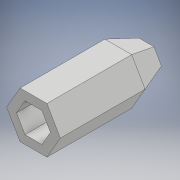
# Autodesk Inventor part: Pieza1
Saved by Autodesk Inventor 2018.2 (Build 222227000, 227)
## iProperties
Created: 2018-01-25
Part Number: Pieza1
Material: Genérico
Document SubType Name: Modeling
Designer: alber
Density: 1 g/cm^3
Appearance: Valor por defecto
Author: alber
Autodesk Inventor part; units mm, degrees
ref_plane "YZ Plane" through (0, 0, 0) normal (1, 0, 0) x (0, 1, 0)
ref_plane "XZ Plane" through (0, 0, 0) normal (0, 1, 0) x (-1, 0, 0)
ref_plane "XY Plane" through (0, 0, 0) normal (0, 0, 1) x (1, 0, 0)
sketch "Boceto16" plane through (0, 0, 0) normal (0, 1, 0) x (-1, 0, 0)
  line L0 (0, 0) -> (6, 0)
  line L1 (6, 0) -> (3, -5.1962)
  line L2 (3, -5.1962) -> (-3, -5.1962)
  line L3 (-3, -5.1962) -> (-6, 0)
  line L4 (-6, 0) -> (-3, 5.1962)
  line L5 (-3, 5.1962) -> (3, 5.1962)
  line L6 (3, 5.1962) -> (6, 0)
  line L7 (6, 0) -> (9.5, 0)
  line L8 (9.5, 0) -> (4.75, -8.2272)
  line L9 (4.75, -8.2272) -> (-4.75, -8.2272)
  line L10 (-4.75, -8.2272) -> (-9.5, 0)
  line L11 (-9.5, 0) -> (-4.75, 8.2272)
  line L12 (-4.75, 8.2272) -> (4.75, 8.2272)
  line L13 (4.75, 8.2272) -> (9.5, 0)
  dimension "d55" = 6
  dimension "d56" = 3.5
  constraints: 28 end point, 2 coincident, 2 horizontal, 26 other
  measures "d55" distance of L0.start L0.end
  measures "d56" distance of L0.end L7.end
extrude "Extrusión10" add sketch "Boceto16" along normal blind 30
sketch "Boceto17" plane through (0, 30, 0) normal (0, 1, 0) x (1, 0, 0)
  line L0 (-9.5, 0) -> (-4.75, -8.2272) projected
  line L1 (-9.5, 0) -> (-4.75, 8.2272)
  line L2 (-4.75, 8.2272) -> (4.75, 8.2272)
  line L3 (4.75, 8.2272) -> (9.5, 0)
  line L4 (9.5, 0) -> (4.75, -8.2272)
  line L5 (4.75, -8.2272) -> (-4.75, -8.2272)
  line L6 (-4.75, -8.2272) -> (-9.5, 0)
  point P0 (0, 0)
  point P1 (0, 0)
  constraints: 12 end point, 1 coincident, 13 other
extrude "Extrusión11" add sketch "Boceto17" along normal blind 10 draft -20
sketch "Boceto18" plane through (0, 40, 0) normal (0, 1, 0) x (1, 0, 0)
  line L0 (0, 1.75) -> (2.1213, 1.75)
  line L1 (0, -1.75) -> (2.1213, -1.75)
  line L2 (0, -1.75) -> (-2.1213, -1.75)
  line L3 (0, 1.75) -> (-2.1213, 1.75)
  arc A0 (-2.1213, 1.75) -> (-2.1213, -1.75) centre (0, 0) ccw
  arc A1 (2.1213, -1.75) -> (2.1213, 1.75) centre (0, 0) ccw
  constraints: 8 end point, 4 point on circle, 2 centre point, 2 coincident, 2 horizontal, 1 parallel
extrude "Extrusión12" cut sketch "Boceto18" against normal blind 5
